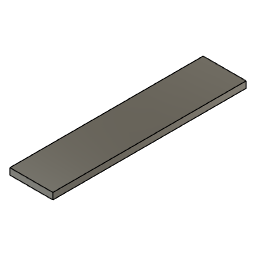
전체 구도 v3 (Autodesk Fusion 360 archive; units mm, degrees)
design "주문컨베이어밸트"
Autodesk Fusion 360 part; units mm, degrees
sketch "스케치1" plane through (0, 0, 0) normal (0, 0, 1) x (1, 0, 0)
  line L0 (-50, 225) -> (50, 225)
  line L1 (50, 225) -> (50, -225)
  line L2 (50, -225) -> (-50, -225)
  line L3 (-50, -225) -> (-50, 225)
  line L4 (0, 225) -> (0, -225) construction
  line L5 (-50, 0) -> (50, 0) construction
  dimension "col" = 100
  dimension "row" = 450
  constraint horizontal L0
  constraint vertical L1
  constraint horizontal L2
  constraint vertical L3
  constraint midpoint L0 L4.start
  constraint midpoint L2 L4.end
  constraint midpoint L3 L5.start
  constraint midpoint L1 L5.end
  constraint midpoint origin L4
  measures "col" distance of L0.start L0.end
  measures "row" distance of L0.end L1.end
extrude "돌출1" add sketch "스케치1" along normal blind 15
equation "height = 15 mm"

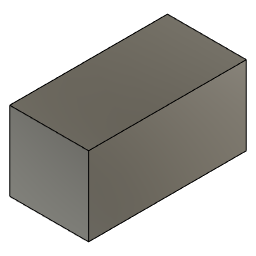
design "피스톤"
Autodesk Fusion 360 part; units mm, degrees
sketch "스케치1" plane through (0, 0, 0) normal (0, 0, 1) x (1, 0, 0)
  line L0 (-25, 50) -> (25, 50)
  line L1 (25, 50) -> (25, -50)
  line L2 (25, -50) -> (-25, -50)
  line L3 (-25, -50) -> (-25, 50)
  line L4 (0, 50) -> (0, -50) construction
  line L5 (25, 0) -> (-25, 0) construction
  dimension "row" = 100
  dimension "col" = 50
  constraint horizontal L0
  constraint vertical L1
  constraint horizontal L2
  constraint vertical L3
  constraint midpoint L0 L4.start
  constraint midpoint L2 L4.end
  constraint midpoint L1 L5.start
  constraint midpoint L3 L5.end
  constraint midpoint L5 origin
  measures "row" distance of L0 L2
  measures "col" distance of L0.start L0.end
extrude "돌출1" add sketch "스케치1" along normal blind 50
equation "height = 50 mm"

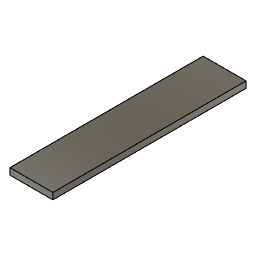
design "분류컨베이어밸트"
Autodesk Fusion 360 part; units mm, degrees
sketch "스케치1" plane through (0, 0, 0) normal (0, 0, 1) x (1, 0, 0)
  line L0 (-50, 225) -> (50, 225)
  line L1 (50, 225) -> (50, -225)
  line L2 (50, -225) -> (-50, -225)
  line L3 (-50, -225) -> (-50, 225)
  line L4 (0, 225) -> (0, -225) construction
  line L5 (-50, 0) -> (50, 0) construction
  dimension "col" = 100
  dimension "row" = 450
  constraint horizontal L0
  constraint vertical L1
  constraint horizontal L2
  constraint vertical L3
  constraint midpoint L0 L4.start
  constraint midpoint L2 L4.end
  constraint midpoint L3 L5.start
  constraint midpoint L1 L5.end
  constraint midpoint origin L4
  measures "col" distance of L0.start L0.end
  measures "row" distance of L0.end L1.end
extrude "돌출1" add sketch "스케치1" along normal blind 15
equation "height = 15 mm"
